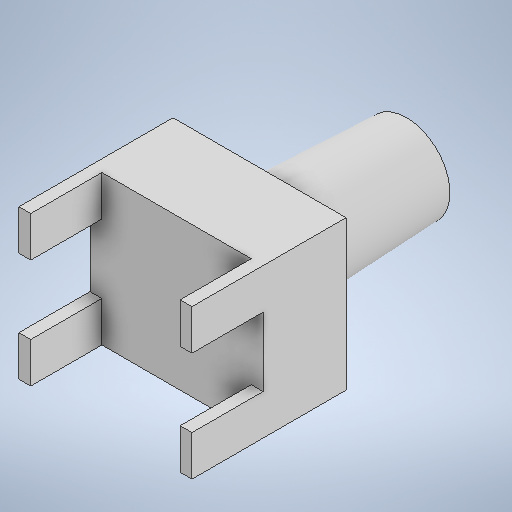
# Autodesk Inventor part: pushbottom3.5mm
Saved by Autodesk Inventor 2025.3 (Build 293356000, 356)
## iProperties
Created: 2025-07-12
Part Number: pushbottom3.5mm
Material: Genérico
Document SubType Name: Modeling
Designer: user
Density: 1 g/cm^3
Appearance: Padrão
Author: user
Autodesk Inventor part; units mm, degrees
ref_plane "YZ Plane" through (0, 0, 0) normal (1, 0, 0) x (0, 1, 0)
ref_plane "XZ Plane" through (0, 0, 0) normal (0, 1, 0) x (-1, 0, 0)
ref_plane "XY Plane" through (0, 0, 0) normal (0, 0, 1) x (1, 0, 0)
sketch "Esboço1" plane through (0, 0, 0) normal (0, 0, 1) x (1, 0, 0)
  line L0 (-3.65, -3.2) -> (3.65, -3.2)
  line L1 (3.65, -3.2) -> (3.65, 3.1)
  line L2 (3.65, 3.1) -> (-3.65, 3.1)
  line L3 (-3.65, 3.1) -> (-3.65, -3.2)
  line L4 (0, 3.1) -> (0, 0)
  dimension "d0" = 7.3
  dimension "d1" = 6.3
  constraints: 10 end point, 2 parallel, 1 horizontal, 1 midpoint, 1 perpendicular, 1 vertical
  measures "d0" distance of L2.end L1.end
  measures "d1" distance of L1.end L0.end
extrude "Extrusão1" add sketch "Esboço1" along normal blind 3.5
sketch "Esboço2" plane through (0, 0, 0) normal (1, 0, 0) x (0, 1, 0)
  line L0 (0, 0) -> (0, -6.2)
  line L1 (0, 0) -> (2.1, 0)
  line L2 (-3.2, 0) -> (3.1, 0) projected
  line L3 (0, -6.2) -> (1.83, -6.2)
  line L4 (1.83, -6.2) -> (2.1, 0)
  dimension "d4" = 6.2
  dimension "d5" = 2.1
  dimension "d6" = 1.83
  constraints: 8 end point, 1 horizontal, 1 point on line, 1 vertical
  measures "d4" distance of L0.start L0.end
  measures "d5" distance of L0.start L1.end
  measures "d6" distance of L0.end L3.end
revolve "Revolução1" add sketch "Esboço2" angle 360 about axis through (0, 0, 0) along (0, 0, -1)
sketch "Esboço3" plane through (0, 0, 3.5) normal (0, 0, 1) x (1, 0, 0)
  line L0 (3.65, 3.1) -> (-3.65, 3.1) projected
  line L1 (3.65, 3.1) -> (3.15, 3.1)
  line L2 (3.15, 3.1) -> (3.15, 1.4)
  line L3 (3.15, 1.4) -> (3.65, 1.4)
  line L4 (3.65, 1.4) -> (3.65, 3.1)
  line L5 (-3.65, -3.2) -> (3.65, -3.2) projected
  line L6 (3.65, -1.5) -> (3.15, -1.5)
  line L7 (3.15, -1.5) -> (3.15, -3.2)
  line L8 (3.15, -3.2) -> (3.65, -3.2)
  line L9 (3.65, -3.2) -> (3.65, -1.5)
  line L10 (-3.15, -1.5) -> (-3.65, -1.5)
  line L11 (-3.65, -1.5) -> (-3.65, -3.2)
  line L12 (-3.65, -3.2) -> (-3.15, -3.2)
  line L13 (-3.15, -3.2) -> (-3.15, -1.5)
  line L14 (-3.65, 3.1) -> (-3.65, -3.2) projected
  line L15 (-3.65, 3.1) -> (-6.7444, 5.2741)
  line L16 (-3.15, 3.1) -> (-3.65, 3.1)
  line L17 (-3.65, 3.1) -> (-3.65, 1.4)
  line L18 (-3.65, 1.4) -> (-3.15, 1.4)
  line L19 (-3.15, 1.4) -> (-3.15, 3.1)
  line L20 (3.65, 3.1) -> (5.0024, 4.4542)
  line L21 (3.65, -3.2) -> (6.7193, -5.088)
  line L22 (-3.65, -3.2) -> (-6.2831, -4.7356)
  point P0 (0, 0)
  point P1 (-3.15, -3.2)
  point P2 (-3.65, 1.4)
  dimension "d8" = 0.5
  dimension "d9" = 1.7
  dimension "d10" = 0.5
  dimension "d11" = 1.7
  dimension "d14" = 0.5
  dimension "d15" = 1.7
  dimension "d19" = 0.5
  dimension "d20" = 1.7
  constraints: 40 end point, 8 parallel, 4 horizontal, 4 perpendicular
  measures "d8" distance of L3.end L2.end
  measures "d9" distance of L2.end L1.end
  measures "d10" distance of L8.end L7.end
  measures "d11" distance of L7.end L6.end
  measures "d14" distance of L12.end L11.end
  measures "d15" distance of L11.end L11.start
  measures "d19" distance of L18.end L18.start
  measures "d20" distance of L18.start L16.end
extrude "Extrusão2" add sketch "Esboço3" along normal blind 3
